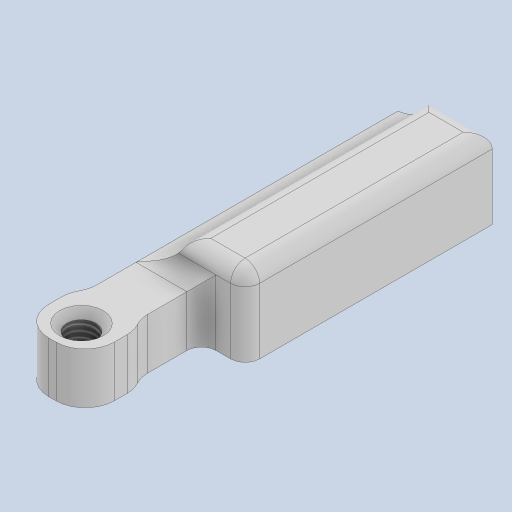
# Autodesk Inventor part: taga1
Saved by Autodesk Inventor 2023 (Build 270158000, 158)
## iProperties
Created: 2022-05-19
Part Number: taga1
Material: Типовые
Document SubType Name: Modeling
Designer: korra
Density: 1 g/cm^3
Appearance: По умолчанию
Author: korra
Autodesk Inventor part; units mm, degrees
ref_plane "YZ Plane" through (0, 0, 0) normal (1, 0, 0) x (0, 1, 0)
sketch "Эскиз1" plane through (0, 0, 0) normal (0, 1, 0) x (-1, 0, 0)
  line L0 (0, 0) -> (3.5, 0)
  line L1 (3.5, 0) -> (3.5, 70)
  line L2 (3.5, 70) -> (0, 70)
  line L3 (0, 70) -> (0, 0)
  dimension "d0" = 3.5
  dimension "d1" = 70
  constraints: 8 end point, 2 parallel, 1 horizontal, 1 perpendicular
  measures "d0" distance of L2.end L1.end
  measures "d1" distance of L0.end L1.end
extrude "Выдавливание1" add sketch "Эскиз1" along normal blind 3.5
sketch "Эскиз2" plane through (0, 3.5, 0) normal (0, 1, 0) x (1, 0, 0)
  line L0 (-3.5, 0) -> (-3.5, -70) projected
  line L1 (-3.5, 0) -> (-3.5, -3)
  line L2 (-3.5, -3) -> (-4, -3)
  line L3 (-4, -3) -> (-4, 0.5)
  line L4 (-4, 0.5) -> (0.5, 0.5)
  line L5 (0.5, 0.5) -> (0.5, -3)
  line L6 (0.5, -3) -> (0, -3)
  line L7 (0, -70) -> (0, 0) projected
  line L8 (0, -3) -> (0, 0)
  line L9 (0, 0) -> (-3.5, 0) projected
  line L10 (0, 0) -> (-3.5, 0)
  line L11 (-3.5, -70) -> (0, -70) projected
  line L12 (0, -70) -> (-3.5, -70)
  line L13 (-3.5, -70) -> (-3.5, -67)
  line L14 (-3.5, -67) -> (-4, -67)
  line L15 (-4, -67) -> (-4, -70.5)
  line L16 (-4, -70.5) -> (0.5, -70.5)
  line L17 (0.5, -70.5) -> (0.5, -67)
  line L18 (0.5, -67) -> (0, -67)
  line L19 (0, -70) -> (0, -67)
  dimension "d6" = 3
  dimension "d7" = 0.5
  dimension "d8" = 3.5
  dimension "d9" = 4.5
  dimension "d10" = 3
  dimension "d11" = 0.5
  dimension "d12" = 3.5
  constraints: 32 end point, 9 perpendicular, 7 point on line, 2 collinear, 1 horizontal
  measures "d6" distance of L0.start L1.end
  measures "d7" distance of L1.end L2.end
  measures "d8" distance of L2.end L3.end
  measures "d9" distance of L3.end L4.end
  measures "d10" distance of L0.end L13.end
  measures "d11" distance of L13.end L14.end
  measures "d12" distance of L14.end L15.end
extrude "Выдавливание2" add sketch "Эскиз2" against normal blind 3.5 contours L0 L2 L3 L4 L5 L6 L7 L9 | L0 L11 L7 L18 L17 L16 L15 L14
sketch "Эскиз3" plane through (0, 3.5, 0) normal (0, 1, 0) x (1, 0, 0)
  line L0 (0, -67) -> (-3.5, -67)
  line L1 (-3.5, -67) -> (-3.5, -70)
  line L2 (-3.5, -70) -> (0, -70)
  line L3 (0, -70) -> (0, -67)
  line L4 (0.5, -67) -> (0, -67) projected
  circle A0 centre (-1.75, -68.5) radius 1
  line L5 (-3.5, -3) -> (0, -3)
  line L6 (0, -3) -> (0, 0)
  line L7 (0, 0) -> (-3.5, 0)
  line L8 (-3.5, 0) -> (-3.5, -3)
  circle A1 centre (-1.75, -1.5) radius 1
  dimension "d15" = 3.5
  dimension "d16" = 3
  dimension "d17" = 0
  dimension "d18" = 2
  dimension "d19" = 3
  dimension "d20" = 2
  constraints: 16 end point, 4 parallel, 2 centre point, 2 horizontal, 2 perpendicular
  measures "d15" distance of L2.end L1.end
  measures "d16" distance of L0.end L1.end
  measures "d17" distance between parallel lines of L4 L0
  measures "d18" diameter of A0
  measures "d19" distance of L6.end L5.end
  measures "d20" diameter of A1
extrude "Выдавливание3" cut sketch "Эскиз3" against normal blind 3.5 contours A0 | A1
chamfer "Фаска1" distance 0.5 angle 45 2 edges at (-2.75, 3.5, 1.5) (-2.75, 3.5, 68.5)
fillet "Сопряжение3" radius 2 6 edges at (-3.5, 1.75, 67) (-4, 1.75, 67) (0, 1.75, 67) (0.5, 1.75, 67) (0.5, 1.75, 70.5) (-4, 1.75, 70.5)
fillet "Сопряжение4" radius 2 6 edges at (0, 1.75, 3) (0.5, 1.75, 3) (0.5, 1.75, -0.5) (-3.5, 1.75, 3) (-4, 1.75, 3) (-4, 1.75, -0.5)
sketch "Эскиз4" plane through (0, 0, 65.6771) normal (1, 0, 0) x (0, 0, -1)
  circle A0 centre (48.6771, 1.75) radius 1
  point P0 (65.6771, 0)
  dimension "d30" = 2
  constraints: 1 centre point
  measures "d30" diameter of A0
extrude "Выдавливание4" cut sketch "Эскиз4" against normal blind 3.5
chamfer "Фаска2" distance 0.5 angle 45 1 edges at (0, 1.75, 18)
sketch "Эскиз5" plane through (0, 0, 65.6771) normal (1, 0, 0) x (0, 0, -1)
  circle A0 centre (48.6771, 1.75) radius 1 projected
  line L0 (0, 3.5) -> (61.3542, 3.5) projected
  line L1 (48.6771, 3.5) -> (50.6771, 3.5)
  line L2 (48.6771, 3.5) -> (46.6771, 3.5)
  line L3 (46.6771, 3.5) -> (46.6771, 4)
  line L4 (46.6771, 4) -> (50.6771, 4)
  line L5 (50.6771, 4) -> (50.6771, 3.5)
  line L6 (0, 0) -> (61.3542, 0) projected
  line L7 (48.6771, 0) -> (50.6771, 0)
  line L8 (48.6771, 0) -> (46.6771, 0)
  line L9 (46.6771, 0) -> (46.6771, -0.5)
  line L10 (46.6771, -0.5) -> (50.6771, -0.5)
  line L11 (50.6771, -0.5) -> (50.6771, 0)
  point P0 (65.6771, 0)
  dimension "d36" = 2
  dimension "d37" = 2
  dimension "d38" = 0.5
  dimension "d39" = 2
  dimension "d40" = 2
  dimension "d41" = 0.5
  constraints: 20 end point, 6 perpendicular, 6 point on line
  measures "d36" distance of L1.start L1.end
  measures "d37" distance of L1.start L2.end
  measures "d38" distance of L2.end L3.end
  measures "d39" distance of L7.start L7.end
  measures "d40" distance of L7.start L8.end
  measures "d41" distance of L8.end L9.end
extrude "Выдавливание5" add sketch "Эскиз5" against normal blind 3.5 contours L3 L4 L5 L0 | L6 L11 L10 L9
fillet "Сопряжение5" radius 2 4 edges at (-1.75, 3.5, 19) (-1.75, 0, 19) (-1.75, 0, 15) (-1.75, 3.5, 15)
fillet "Сопряжение6" radius 2 4 edges at (-1.75, 4, 15) (-1.75, 4, 19) (-1.75, -0.5, 15) (-1.75, -0.5, 19)
thread "Резьба1" size "M2x0.4" class "6H" standard "ANSI Metric M Profile" full length
thread "Резьба2" size "M2x0.4" class "6H" standard "ANSI Metric M Profile" full length
thread "Резьба3" size "M2x0.4" class "6H" standard "ANSI Metric M Profile" full length
ref_plane "РабПлоскость1" through (0, 3.3, 65.6771) normal (1, 0, 0) x (0, 0, -1)
sketch "Эскиз8" plane through (0, 3.3, 65.6771) normal (1, 0, 0) x (0, 0, -1)
  line L0 (22.677, 14.6701) -> (92.4847, 14.6701)
  line L1 (92.4847, 14.6701) -> (92.4847, -32.0033)
  line L2 (92.4847, -32.0033) -> (22.677, -32.0033)
  line L3 (22.677, -32.0033) -> (22.677, 14.6701)
  line L4 (0, 0) -> (0, 0.2) projected
  point P0 (65.6771, -3.3)
  dimension "d67" = 22.677
  constraints: 8 end point, 2 parallel, 1 horizontal, 1 perpendicular
  measures "d67" distance between parallel lines of L3 L4
extrude "Выдавливание8" cut sketch "Эскиз8" against normal blind 10
sketch "Эскиз9" plane through (0, 3.3, 65.6771) normal (-1, 0, 0) x (0, 0, 1)
  circle A0 centre (-75.9326, -18.5571) radius 43.8023
  point P0 (-65.6771, -3.3)
  constraints: 1 centre point
extrude "Выдавливание9" cut sketch "Эскиз9" against normal blind 10
ref_plane "РабПлоскость2" through (0, 0.2, 43.0001) normal (0, 0, -1) x (-1, 0, 0)
sketch "Эскиз11" plane through (0, 0.2, 43.0001) normal (0, 0, -1) x (-1, 0, 0)
  line L0 (7.9005, -2.3763) -> (-11.0516, -2.3763)
  line L1 (-11.0516, -2.3763) -> (-11.0516, 8.596)
  line L2 (-11.0516, 8.596) -> (7.9005, 8.596)
  line L3 (7.9005, 8.596) -> (7.9005, -2.3763)
  point P0 (0, -0.2)
  constraints: 8 end point, 2 parallel, 1 horizontal, 1 perpendicular
extrude "Выдавливание11" cut sketch "Эскиз11" against normal blind 2
sketch "Эскиз12" plane through (0, 0.2, 45.0001) normal (0, 0, -1) x (-1, 0, 0)
  line L0 (0, -0.2) -> (-3, -0.2)
  line L1 (-3, -0.2) -> (-3, 3.3)
  line L2 (-3, 3.3) -> (0, 3.3)
  line L3 (0, 3.3) -> (0, -0.2)
  dimension "d79" = 3
  constraints: 8 end point, 2 parallel, 1 horizontal, 1 perpendicular
  measures "d79" distance of L1.end L2.end
extrude "Выдавливание12" add sketch "Эскиз12" against normal blind 17
sketch "Эскиз13" plane through (0, 3.5, 0) normal (0, 1, 0) x (1, 0, 0)
  line L0 (3, -45.0001) -> (3, -62.0001) projected
  line L1 (3, -62.0001) -> (0, -62.0001) projected
  line L2 (3, -45.0001) -> (3, -62.0001)
  line L3 (3, -62.0001) -> (0, -62.0001)
  line L4 (0, -62.0001) -> (-1, -62.0001)
  line L5 (-1, -62.0001) -> (-1, -45.0001)
  line L6 (-3.5, -45.0001) -> (3, -45.0001) projected
  line L7 (3, -45.0001) -> (-1, -45.0001)
  point P0 (0, 0)
  dimension "d82" = 1
  constraints: 10 end point, 3 perpendicular, 2 point on line, 1 vertical
  measures "d82" distance of L1.end L4.end
extrude "Выдавливание13" add sketch "Эскиз13" along normal blind 2
sketch "Эскиз15" plane through (0, 0.2, 45.0001) normal (0, 0, -1) x (-1, 0, 0)
  circle A0 centre (-0.5, 2.55) radius 1.425
  line L0 (-3, 5.3) -> (1, 5.3) projected
  line L1 (-3, 5.3) -> (-3, -0.2) projected
  point P0 (0, -0.2)
  point P1 (-1, 5.3)
  point P2 (-3, -1.2)
  dimension "d87" = 2.85
  dimension "d88" = 2.75
  dimension "d89" = 2.5
  constraints: 1 centre point, 1 midpoint
  measures "d87" diameter of A0
  measures "d88" vertical distance of point (-1, 5.3) A0.centre
  measures "d89" distance from line of L1 A0.centre
extrude "Выдавливание15" cut sketch "Эскиз15" against normal blind 15
fillet "Сопряжение18" radius 3 1 edges at (-1, 3.5, 53.5001)
fillet "Сопряжение19" radius 1 4 edges at (-1, 5.5, 53.5001) (1, 5.5, 45.0001) (3, 5.5, 53.5001) (1, 5.5, 62.0001)
fillet "Сопряжение20" radius 1 3 edges at (0, 1.75, 62.0001) (2.7071, 5.2071, 61.7072) (3, 2.25, 62.0001)
fillet "Сопряжение21" radius 1 1 edges at (-1.25, 3.5, 62.0001)
